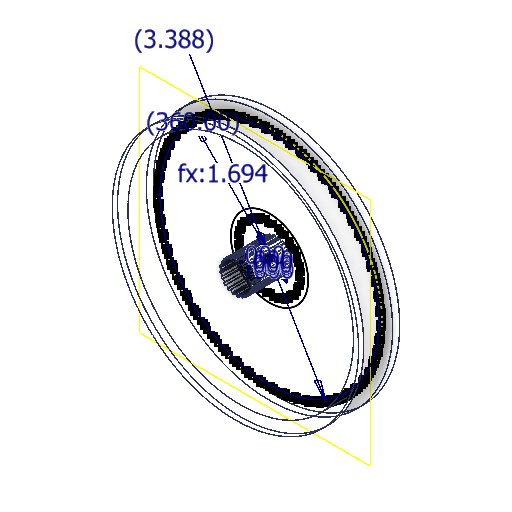
# Autodesk Inventor part: Diff Large Pulley
Saved by Autodesk Inventor 2025.2 (Build 292293000, 293)
## iProperties
Created: 2025-02-20
Part Number: Diff Large Pulley
Material: Generic
Document SubType Name: Modeling
Designer: Jakeg
Density: 1 g/cm^3
Appearance: PTFE
Author: Jakeg
Autodesk Inventor part; units mm, degrees
(part 1 of 2)
ref_plane "YZ Plane" through (0, 0, 0) normal (1, 0, 0) x (0, 1, 0)
ref_plane "XZ Plane" through (0, 0, 0) normal (0, 1, 0) x (-1, 0, 0)
ref_plane "XY Plane" through (0, 0, 0) normal (0, 0, 1) x (1, 0, 0)
sketch "Sketch1" plane through (0, 0, 0) normal (0, 0, 1) x (1, 0, 0)
  circle A0 centre (0, 0) radius 46.99
  dimension "d0" = 93.98
  constraints: 1 centre point, 1 coincident
  measures "d0" diameter of A0
extrude "Extrusion1" add sketch "Sketch1" along normal blind 15.7
ref_plane "Work Plane1" through (0, 0, 8.2) normal (0, 0, 1) x (1, 0, 0)
sketch "Sketch2" plane through (0, 0, 8.2) normal (0, 0, 1) x (1, 0, 0)
  circle A0 centre (0, 0) radius 43.0276
  circle A1 centre (0, 0) radius 46.99
  dimension "d4" = 86.0552
  dimension "d39" = 93.98
  constraints: 2 centre point, 2 coincident
  measures "d4" diameter of A0
  measures "d39" diameter of A1
extrude "Extrusion2" cut sketch "Sketch2" along normal mid plane 11
sketch "Sketch3" plane through (0, 0, 15.7) normal (0, 0, 1) x (1, 0, 0)
  circle A0 centre (0, 0) radius 6
  circle A1 centre (0, 20.32) radius 3.175
  circle A2 centre (0, -20.32) radius 3.175
  dimension "d7" = 12
  dimension "d13" = 6.35
  dimension "d14" = 20.32
  dimension "d15" = 6.35
  dimension "d16" = 20.32
  constraints: 3 centre point, 1 coincident
  measures "d7" diameter of A0
  measures "d13" diameter of A1
  measures "d14" distance of point (0, 0) A1.centre
  measures "d15" diameter of A2
  measures "d16" distance of point (0, 0) A2.centre
extrude "Extrusion3" cut sketch "Sketch3" against normal through all contours A0
sketch "Sketch5" plane through (0, 0, 15.7) normal (0, 0, 1) x (1, 0, 0)
  circle A0 centre (0, 0) radius 6 projected
  arc A1 (-1.2778, -5.5469) -> (-2.2267, -5.2386) centre (-1.8274, -5.6241) ccw
  arc A2 (-1.2783, -5.8289) -> (-1.2778, -5.5469) centre (-2.2681, -5.6859) ccw
  arc A3 (-1.2783, -5.8289) -> (-1.1583, -5.9977) centre (-1.1299, -5.8504) ccw
  arc A4 (-1.1583, -5.9977) -> (-0.7518, -6.0621) centre (0, 0) ccw
  arc A5 (-0.7518, -6.0621) -> (-0.5855, -5.9387) centre (-0.7333, -5.9132) ccw
  arc A6 (-0.4989, -5.6703) -> (-0.5855, -5.9387) centre (0.4, -6.1085) ccw
  arc A7 (0.4989, -5.6703) -> (-0.4989, -5.6703) centre (0, -5.9135) ccw
  arc A8 (0.5855, -5.9387) -> (0.4989, -5.6703) centre (-0.4, -6.1085) ccw
  arc A9 (0.5855, -5.9387) -> (0.7518, -6.0621) centre (0.7333, -5.9132) ccw
  arc A10 (0.7518, -6.0621) -> (1.1583, -5.9977) centre (0, 0) ccw
  arc A11 (1.1583, -5.9977) -> (1.2783, -5.8289) centre (1.1299, -5.8504) ccw
  arc A12 (1.2778, -5.5469) -> (1.2783, -5.8289) centre (2.2681, -5.6859) ccw
  arc A13 (2.2267, -5.2386) -> (1.2778, -5.5469) centre (1.8274, -5.6241) ccw
  arc A14 (2.392, -5.4671) -> (2.2267, -5.2386) centre (1.5072, -5.9331) ccw
  arc A15 (2.392, -5.4671) -> (2.5882, -5.5331) centre (2.5247, -5.3972) ccw
  arc A16 (2.5882, -5.5331) -> (2.955, -5.3462) centre (0, 0) ccw
  arc A17 (2.955, -5.3462) -> (3.017, -5.1486) centre (2.8824, -5.2149) ccw
  arc A18 (2.9293, -4.8806) -> (3.017, -5.1486) centre (3.9141, -4.7068) ccw
  arc A19 (3.7365, -4.2941) -> (2.9293, -4.8806) centre (3.4759, -4.7841) ccw
  arc A20 (3.9643, -4.4604) -> (3.7365, -4.2941) centre (3.2669, -5.177) ccw
  arc A21 (3.9643, -4.4604) -> (4.1714, -4.4624) centre (4.0689, -4.3529) ccw
  arc A22 (4.1714, -4.4624) -> (4.4624, -4.1714) centre (0, 0) ccw
  arc A23 (4.4624, -4.1714) -> (4.4604, -3.9643) centre (4.3529, -4.0689) ccw
  arc A24 (4.2941, -3.7365) -> (4.4604, -3.9643) centre (5.177, -3.2669) ccw
  arc A25 (4.8806, -2.9293) -> (4.2941, -3.7365) centre (4.7841, -3.4759) ccw
  arc A26 (5.1486, -3.017) -> (4.8806, -2.9293) centre (4.7068, -3.9141) ccw
  arc A27 (5.1486, -3.017) -> (5.3462, -2.955) centre (5.2149, -2.8824) ccw
  arc A28 (5.3462, -2.955) -> (5.5331, -2.5882) centre (0, 0) ccw
  arc A29 (5.5331, -2.5882) -> (5.4671, -2.392) centre (5.3972, -2.5247) ccw
  arc A30 (5.2386, -2.2267) -> (5.4671, -2.392) centre (5.9331, -1.5072) ccw
  arc A31 (5.5469, -1.2778) -> (5.2386, -2.2267) centre (5.6241, -1.8274) ccw
  arc A32 (5.8289, -1.2783) -> (5.5469, -1.2778) centre (5.6859, -2.2681) ccw
  arc A33 (5.8289, -1.2783) -> (5.9977, -1.1583) centre (5.8504, -1.1299) ccw
  arc A34 (5.9977, -1.1583) -> (6.0621, -0.7518) centre (0, 0) ccw
  arc A35 (6.0621, -0.7518) -> (5.9387, -0.5855) centre (5.9132, -0.7333) ccw
  arc A36 (5.6703, -0.4989) -> (5.9387, -0.5855) centre (6.1085, 0.4) ccw
  arc A37 (5.6703, 0.4989) -> (5.6703, -0.4989) centre (5.9135, 0) ccw
  arc A38 (5.9387, 0.5855) -> (5.6703, 0.4989) centre (6.1085, -0.4) ccw
  arc A39 (5.9387, 0.5855) -> (6.0621, 0.7518) centre (5.9132, 0.7333) ccw
  arc A40 (6.0621, 0.7518) -> (5.9977, 1.1583) centre (0, 0) ccw
  arc A41 (5.9977, 1.1583) -> (5.8289, 1.2783) centre (5.8504, 1.1299) ccw
  arc A42 (5.5469, 1.2778) -> (5.8289, 1.2783) centre (5.6859, 2.2681) ccw
  arc A43 (5.2386, 2.2267) -> (5.5469, 1.2778) centre (5.6241, 1.8274) ccw
  arc A44 (5.4671, 2.392) -> (5.2386, 2.2267) centre (5.9331, 1.5072) ccw
  arc A45 (5.4671, 2.392) -> (5.5331, 2.5882) centre (5.3972, 2.5247) ccw
  arc A46 (5.5331, 2.5882) -> (5.3462, 2.955) centre (0, 0) ccw
  arc A47 (5.3462, 2.955) -> (5.1486, 3.017) centre (5.2149, 2.8824) ccw
  arc A48 (4.8806, 2.9293) -> (5.1486, 3.017) centre (4.7068, 3.9141) ccw
  arc A49 (4.2941, 3.7365) -> (4.8806, 2.9293) centre (4.7841, 3.4759) ccw
  arc A50 (4.4604, 3.9643) -> (4.2941, 3.7365) centre (5.177, 3.2669) ccw
  arc A51 (4.4604, 3.9643) -> (4.4624, 4.1714) centre (4.3529, 4.0689) ccw
  arc A52 (4.4624, 4.1714) -> (4.1714, 4.4624) centre (0, 0) ccw
  arc A53 (4.1714, 4.4624) -> (3.9643, 4.4604) centre (4.0689, 4.3529) ccw
  arc A54 (3.7365, 4.2941) -> (3.9643, 4.4604) centre (3.2669, 5.177) ccw
  arc A55 (2.9293, 4.8806) -> (3.7365, 4.2941) centre (3.4759, 4.7841) ccw
  arc A56 (3.017, 5.1486) -> (2.9293, 4.8806) centre (3.9141, 4.7068) ccw
  arc A57 (3.017, 5.1486) -> (2.955, 5.3462) centre (2.8824, 5.2149) ccw
  arc A58 (2.955, 5.3462) -> (2.5882, 5.5331) centre (0, 0) ccw
  arc A59 (2.5882, 5.5331) -> (2.392, 5.4671) centre (2.5247, 5.3972) ccw
  arc A60 (2.2267, 5.2386) -> (2.392, 5.4671) centre (1.5072, 5.9331) ccw
  arc A61 (1.2778, 5.5469) -> (2.2267, 5.2386) centre (1.8274, 5.6241) ccw
  arc A62 (1.2783, 5.8289) -> (1.2778, 5.5469) centre (2.2681, 5.6859) ccw
  arc A63 (1.2783, 5.8289) -> (1.1583, 5.9977) centre (1.1299, 5.8504) ccw
  arc A64 (1.1583, 5.9977) -> (0.7518, 6.0621) centre (0, 0) ccw
  arc A65 (0.7518, 6.0621) -> (0.5855, 5.9387) centre (0.7333, 5.9132) ccw
  arc A66 (0.4989, 5.6703) -> (0.5855, 5.9387) centre (-0.4, 6.1085) ccw
  arc A67 (-0.4989, 5.6703) -> (0.4989, 5.6703) centre (0, 5.9135) ccw
  arc A68 (-0.5855, 5.9387) -> (-0.4989, 5.6703) centre (0.4, 6.1085) ccw
  arc A69 (-0.5855, 5.9387) -> (-0.7518, 6.0621) centre (-0.7333, 5.9132) ccw
  arc A70 (-0.7518, 6.0621) -> (-1.1583, 5.9977) centre (0, 0) ccw
  arc A71 (-1.1583, 5.9977) -> (-1.2783, 5.8289) centre (-1.1299, 5.8504) ccw
  arc A72 (-1.2778, 5.5469) -> (-1.2783, 5.8289) centre (-2.2681, 5.6859) ccw
  arc A73 (-2.2267, 5.2386) -> (-1.2778, 5.5469) centre (-1.8274, 5.6241) ccw
  arc A74 (-2.392, 5.4671) -> (-2.2267, 5.2386) centre (-1.5072, 5.9331) ccw
  arc A75 (-2.392, 5.4671) -> (-2.5882, 5.5331) centre (-2.5247, 5.3972) ccw
  arc A76 (-2.5882, 5.5331) -> (-2.955, 5.3462) centre (0, 0) ccw
  arc A77 (-2.955, 5.3462) -> (-3.017, 5.1486) centre (-2.8824, 5.2149) ccw
  arc A78 (-2.9293, 4.8806) -> (-3.017, 5.1486) centre (-3.9141, 4.7068) ccw
  arc A79 (-3.7365, 4.2941) -> (-2.9293, 4.8806) centre (-3.4759, 4.7841) ccw
  arc A80 (-3.9643, 4.4604) -> (-3.7365, 4.2941) centre (-3.2669, 5.177) ccw
  arc A81 (-3.9643, 4.4604) -> (-4.1714, 4.4624) centre (-4.0689, 4.3529) ccw
  arc A82 (-4.1714, 4.4624) -> (-4.4624, 4.1714) centre (0, 0) ccw
  arc A83 (-4.4624, 4.1714) -> (-4.4604, 3.9643) centre (-4.3529, 4.0689) ccw
  arc A84 (-4.2941, 3.7365) -> (-4.4604, 3.9643) centre (-5.177, 3.2669) ccw
  arc A85 (-4.8806, 2.9293) -> (-4.2941, 3.7365) centre (-4.7841, 3.4759) ccw
  arc A86 (-5.1486, 3.017) -> (-4.8806, 2.9293) centre (-4.7068, 3.9141) ccw
  arc A87 (-5.1486, 3.017) -> (-5.3462, 2.955) centre (-5.2149, 2.8824) ccw
  arc A88 (-5.3462, 2.955) -> (-5.5331, 2.5882) centre (0, 0) ccw
  arc A89 (-5.5331, 2.5882) -> (-5.4671, 2.392) centre (-5.3972, 2.5247) ccw
  arc A90 (-5.2386, 2.2267) -> (-5.4671, 2.392) centre (-5.9331, 1.5072) ccw
  arc A91 (-5.5469, 1.2778) -> (-5.2386, 2.2267) centre (-5.6241, 1.8274) ccw
  arc A92 (-5.8289, 1.2783) -> (-5.5469, 1.2778) centre (-5.6859, 2.2681) ccw
  arc A93 (-5.8289, 1.2783) -> (-5.9977, 1.1583) centre (-5.8504, 1.1299) ccw
  arc A94 (-5.9977, 1.1583) -> (-6.0621, 0.7518) centre (0, 0) ccw
  arc A95 (-6.0621, 0.7518) -> (-5.9387, 0.5855) centre (-5.9132, 0.7333) ccw
  arc A96 (-5.6703, 0.4989) -> (-5.9387, 0.5855) centre (-6.1085, -0.4) ccw
  arc A97 (-5.6703, -0.4989) -> (-5.6703, 0.4989) centre (-5.9135, 0) ccw
  arc A98 (-5.9387, -0.5855) -> (-5.6703, -0.4989) centre (-6.1085, 0.4) ccw
  arc A99 (-5.9387, -0.5855) -> (-6.0621, -0.7518) centre (-5.9132, -0.7333) ccw
  arc A100 (-6.0621, -0.7518) -> (-5.9977, -1.1583) centre (0, 0) ccw
  arc A101 (-5.9977, -1.1583) -> (-5.8289, -1.2783) centre (-5.8504, -1.1299) ccw
  arc A102 (-5.5469, -1.2778) -> (-5.8289, -1.2783) centre (-5.6859, -2.2681) ccw
  arc A103 (-5.2386, -2.2267) -> (-5.5469, -1.2778) centre (-5.6241, -1.8274) ccw
  arc A104 (-5.4671, -2.392) -> (-5.2386, -2.2267) centre (-5.9331, -1.5072) ccw
  arc A105 (-5.4671, -2.392) -> (-5.5331, -2.5882) centre (-5.3972, -2.5247) ccw
  arc A106 (-5.5331, -2.5882) -> (-5.3462, -2.955) centre (0, 0) ccw
  arc A107 (-5.3462, -2.955) -> (-5.1486, -3.017) centre (-5.2149, -2.8824) ccw
  arc A108 (-4.8806, -2.9293) -> (-5.1486, -3.017) centre (-4.7068, -3.9141) ccw
  arc A109 (-4.2941, -3.7365) -> (-4.8806, -2.9293) centre (-4.7841, -3.4759) ccw
  arc A110 (-4.4604, -3.9643) -> (-4.2941, -3.7365) centre (-5.177, -3.2669) ccw
  arc A111 (-4.4604, -3.9643) -> (-4.4624, -4.1714) centre (-4.3529, -4.0689) ccw
  arc A112 (-4.4624, -4.1714) -> (-4.1714, -4.4624) centre (0, 0) ccw
  arc A113 (-4.1714, -4.4624) -> (-3.9643, -4.4604) centre (-4.0689, -4.3529) ccw
  arc A114 (-3.7365, -4.2941) -> (-3.9643, -4.4604) centre (-3.2669, -5.177) ccw
  arc A115 (-2.9293, -4.8806) -> (-3.7365, -4.2941) centre (-3.4759, -4.7841) ccw
  arc A116 (-3.017, -5.1486) -> (-2.9293, -4.8806) centre (-3.9141, -4.7068) ccw
  arc A117 (-3.017, -5.1486) -> (-2.955, -5.3462) centre (-2.8824, -5.2149) ccw
  arc A118 (-2.955, -5.3462) -> (-2.5882, -5.5331) centre (0, 0) ccw
  arc A119 (-2.5882, -5.5331) -> (-2.392, -5.4671) centre (-2.5247, -5.3972) ccw
  arc A120 (-2.2267, -5.2386) -> (-2.392, -5.4671) centre (-1.5072, -5.9331) ccw
  point P0 (-3.9904, -4.4807)
  point P1 (-3.0283, -5.1797)
  point P2 (-5.1797, -3.0283)
  point P3 (-4.4807, -3.9904)
  point P4 (-5.862, -1.2794)
  point P5 (-5.4945, -2.4105)
  point P6 (-5.9705, 0.5947)
  point P7 (-5.9705, -0.5947)
  point P8 (-5.4945, 2.4105)
  point P9 (-5.862, 1.2794)
  point P10 (-4.4807, 3.9904)
  point P11 (-5.1797, 3.0283)
  point P12 (-3.0283, 5.1797)
  point P13 (-3.9904, 4.4807)
  point P14 (-1.2794, 5.862)
  point P15 (-2.4105, 5.4945)
  point P16 (0.5947, 5.9705)
  point P17 (-0.5947, 5.9705)
  point P18 (2.4105, 5.4945)
  point P19 (1.2794, 5.862)
  point P20 (3.9904, 4.4807)
  point P21 (3.0283, 5.1797)
  point P22 (5.1797, 3.0283)
  point P23 (4.4807, 3.9904)
  point P24 (5.862, 1.2794)
  point P25 (5.4945, 2.4105)
  point P26 (5.9705, -0.5947)
  point P27 (5.9705, 0.5947)
  point P28 (5.4945, -2.4105)
  point P29 (5.862, -1.2794)
  point P30 (4.4807, -3.9904)
  point P31 (5.1797, -3.0283)
  point P32 (3.0283, -5.1797)
  point P33 (3.9904, -4.4807)
  point P34 (1.2794, -5.862)
  point P35 (2.4105, -5.4945)
  point P36 (-0.5947, -5.9705)
  point P37 (0.5947, -5.9705)
  point P38 (-2.4105, -5.4945)
  point P39 (-1.2794, -5.862)
  dimension "d21" = 0
  dimension "d22" = 0
  constraints: 240 point on circle, 120 centre point, 1 coincident, 1 other
  measures "d21" distance of point (0, 0) A4.centre
  measures "d22" distance of A4.centre point (0, 0)
extrude "Extrusion5" add sketch "Sketch5" against normal blind 15.7 contours A0 A35 A36 A37 A38 A39 | A0 A41 A40 A39 | A35 A34 A33 A0 | A41 A42 A43 A44 A45 A0 | A0 A29 A30 A31 A32 A33 | A0 A47 A46 A45 | A29 A28 A27 A0 | A47 A48 A49 A50 A51 A0 | A0 A23 A24 A25 A26 A27 | A0 A53 A52 A51 | A23 A22 A21 A0 | A53 A54 A55 A56 A57 A0 | A0 A17 A18 A19 A20 A21 | A0 A59 A58 A57 | A17 A16 A15 A0 | A59 A60 A61 A62 A63 A0 | A0 A11 A12 A13 A14 A15 | A0 A65 A64 A63 | A11 A10 A9 A0 | A65 A66 A67 A68 A69 A0 | A0 A5 A6 A7 A8 A9 | A0 A71 A70 A69 | A5 A4 A3 A0 | A71 A72 A73 A74 A75 A0 | A0 A119 A120 A1 A2 A3 | A0 A77 A76 A75 | A119 A118 A117 A0 | A77 A78 A79 A80 A81 A0 | A0 A113 A114 A115 A116 A117 | A0 A83 A82 A81 | A113 A112 A111 A0 | A83 A84 A85 A86 A87 A0 | A0 A107 A108 A109 A110 A111 | A0 A89 A88 A87 | A107 A106 A105 A0 | A89 A90 A91 A92 A93 A0 | A0 A101 A102 A103 A104 A105 | A0 A95 A94 A93 | A101 A100 A99 A0 | A95 A96 A97 A98 A99 A0
sketch "Sketch8" plane through (0, 0, 2.7) normal (0, 0, 1) x (1, 0, 0)
  circle A0 centre (0, 0) radius 14.7498
  line L0 (3.5809, 11.7957) -> (3.627, 10.7394)
  arc A1 (3.627, 10.7394) -> (3.7836, 10.5159) centre (3.8808, 10.7505) ccw
  line L1 (3.7836, 10.5159) -> (4.7604, 10.1112)
  arc A2 (4.7604, 10.1112) -> (5.0292, 10.1586) centre (4.8576, 10.3459) ccw
  line L2 (5.0292, 10.1586) -> (5.8087, 10.8729)
  arc A3 (6.1044, 10.9073) -> (5.8087, 10.8729) centre (5.9803, 10.6856) ccw
  arc A4 (7.741, 9.8138) -> (6.1044, 10.9073) centre (0, 0) ccw
  arc A5 (7.8223, 9.5275) -> (7.741, 9.8138) centre (7.5837, 9.6143) ccw
  line L3 (7.8223, 9.5275) -> (7.4607, 8.534)
  arc A6 (7.4607, 8.534) -> (7.5198, 8.2675) centre (7.6994, 8.4471) ccw
  line L4 (7.5198, 8.2675) -> (8.2675, 7.5198)
  arc A7 (8.2675, 7.5198) -> (8.534, 7.4607) centre (8.4471, 7.6994) ccw
  line L5 (8.534, 7.4607) -> (9.5275, 7.8223)
  arc A8 (9.8138, 7.741) -> (9.5275, 7.8223) centre (9.6143, 7.5837) ccw
  arc A9 (10.9073, 6.1044) -> (9.8138, 7.741) centre (0, 0) ccw
  arc A10 (10.8729, 5.8087) -> (10.9073, 6.1044) centre (10.6856, 5.9803) ccw
  line L6 (10.8729, 5.8087) -> (10.1586, 5.0292)
  arc A11 (10.1586, 5.0292) -> (10.1112, 4.7604) centre (10.3459, 4.8576) ccw
  line L7 (10.1112, 4.7604) -> (10.5159, 3.7836)
  arc A12 (10.5159, 3.7836) -> (10.7394, 3.627) centre (10.7505, 3.8808) ccw
  line L8 (10.7394, 3.627) -> (11.7957, 3.5809)
  arc A13 (12.0291, 3.3962) -> (11.7957, 3.5809) centre (11.7846, 3.3271) ccw
  arc A14 (12.4131, 1.4657) -> (12.0291, 3.3962) centre (0, 0) ccw
  arc A15 (12.2682, 1.2057) -> (12.4131, 1.4657) centre (12.1608, 1.4359) ccw
  line L9 (12.2682, 1.2057) -> (11.31, 0.7589)
  arc A16 (11.31, 0.7589) -> (11.1633, 0.5287) centre (11.4173, 0.5287) ccw
  line L10 (11.1633, 0.5287) -> (11.1633, -0.5287)
  arc A17 (11.1633, -0.5287) -> (11.31, -0.7589) centre (11.4173, -0.5287) ccw
  line L11 (11.31, -0.7589) -> (12.2682, -1.2057)
  arc A18 (12.4131, -1.4657) -> (12.2682, -1.2057) centre (12.1608, -1.4359) ccw
  arc A19 (12.0291, -3.3962) -> (12.4131, -1.4657) centre (0, 0) ccw
  arc A20 (11.7957, -3.5809) -> (12.0291, -3.3962) centre (11.7846, -3.3271) ccw
  line L12 (11.7957, -3.5809) -> (10.7394, -3.627)
  arc A21 (10.7394, -3.627) -> (10.5159, -3.7836) centre (10.7505, -3.8808) ccw
  line L13 (10.5159, -3.7836) -> (10.1112, -4.7604)
  arc A22 (10.1112, -4.7604) -> (10.1586, -5.0292) centre (10.3459, -4.8576) ccw
  line L14 (10.1586, -5.0292) -> (10.8729, -5.8087)
  arc A23 (10.9073, -6.1044) -> (10.8729, -5.8087) centre (10.6856, -5.9803) ccw
  arc A24 (9.8138, -7.741) -> (10.9073, -6.1044) centre (0, 0) ccw
  arc A25 (9.5275, -7.8223) -> (9.8138, -7.741) centre (9.6143, -7.5837) ccw
  line L15 (9.5275, -7.8223) -> (8.534, -7.4607)
  arc A26 (8.534, -7.4607) -> (8.2675, -7.5198) centre (8.4471, -7.6994) ccw
  line L16 (8.2675, -7.5198) -> (7.5198, -8.2675)
  arc A27 (7.5198, -8.2675) -> (7.4607, -8.534) centre (7.6994, -8.4471) ccw
  line L17 (7.4607, -8.534) -> (7.8223, -9.5275)
  arc A28 (7.741, -9.8138) -> (7.8223, -9.5275) centre (7.5837, -9.6143) ccw
  arc A29 (6.1044, -10.9073) -> (7.741, -9.8138) centre (0, 0) ccw
  arc A30 (5.8087, -10.8729) -> (6.1044, -10.9073) centre (5.9803, -10.6856) ccw
  line L18 (5.8087, -10.8729) -> (5.0292, -10.1586)
  arc A31 (5.0292, -10.1586) -> (4.7604, -10.1112) centre (4.8576, -10.3459) ccw
  line L19 (4.7604, -10.1112) -> (3.7836, -10.5159)
  arc A32 (3.7836, -10.5159) -> (3.627, -10.7394) centre (3.8808, -10.7505) ccw
  line L20 (3.627, -10.7394) -> (3.5809, -11.7957)
  arc A33 (3.3962, -12.0291) -> (3.5809, -11.7957) centre (3.3271, -11.7846) ccw
  arc A34 (1.4657, -12.4131) -> (3.3962, -12.0291) centre (0, 0) ccw
  arc A35 (1.2057, -12.2682) -> (1.4657, -12.4131) centre (1.4359, -12.1608) ccw
  line L21 (1.2057, -12.2682) -> (0.7589, -11.31)
  arc A36 (0.7589, -11.31) -> (0.5287, -11.1633) centre (0.5287, -11.4173) ccw
  line L22 (0.5287, -11.1633) -> (-0.5287, -11.1633)
  arc A37 (-0.5287, -11.1633) -> (-0.7589, -11.31) centre (-0.5287, -11.4173) ccw
  line L23 (-0.7589, -11.31) -> (-1.2057, -12.2682)
  arc A38 (-1.4657, -12.4131) -> (-1.2057, -12.2682) centre (-1.4359, -12.1608) ccw
  arc A39 (-3.3962, -12.0291) -> (-1.4657, -12.4131) centre (0, 0) ccw
  arc A40 (-3.5809, -11.7957) -> (-3.3962, -12.0291) centre (-3.3271, -11.7846) ccw
  line L24 (-3.5809, -11.7957) -> (-3.627, -10.7394)
  arc A41 (-3.627, -10.7394) -> (-3.7836, -10.5159) centre (-3.8808, -10.7505) ccw
  line L25 (-3.7836, -10.5159) -> (-4.7604, -10.1112)
  arc A42 (-4.7604, -10.1112) -> (-5.0292, -10.1586) centre (-4.8576, -10.3459) ccw
  line L26 (-5.0292, -10.1586) -> (-5.8087, -10.8729)
  arc A43 (-6.1044, -10.9073) -> (-5.8087, -10.8729) centre (-5.9803, -10.6856) ccw
  arc A44 (-7.741, -9.8138) -> (-6.1044, -10.9073) centre (0, 0) ccw
  arc A45 (-7.8223, -9.5275) -> (-7.741, -9.8138) centre (-7.5837, -9.6143) ccw
  line L27 (-7.8223, -9.5275) -> (-7.4607, -8.534)
  arc A46 (-7.4607, -8.534) -> (-7.5198, -8.2675) centre (-7.6994, -8.4471) ccw
  line L28 (-7.5198, -8.2675) -> (-8.2675, -7.5198)
  arc A47 (-8.2675, -7.5198) -> (-8.534, -7.4607) centre (-8.4471, -7.6994) ccw
  line L29 (-8.534, -7.4607) -> (-9.5275, -7.8223)
  arc A48 (-9.8138, -7.741) -> (-9.5275, -7.8223) centre (-9.6143, -7.5837) ccw
  arc A49 (-10.9073, -6.1044) -> (-9.8138, -7.741) centre (0, 0) ccw
  arc A50 (-10.8729, -5.8087) -> (-10.9073, -6.1044) centre (-10.6856, -5.9803) ccw
  line L30 (-10.8729, -5.8087) -> (-10.1586, -5.0292)
  arc A51 (-10.1586, -5.0292) -> (-10.1112, -4.7604) centre (-10.3459, -4.8576) ccw
  line L31 (-10.1112, -4.7604) -> (-10.5159, -3.7836)
  arc A52 (-10.5159, -3.7836) -> (-10.7394, -3.627) centre (-10.7505, -3.8808) ccw
  line L32 (-10.7394, -3.627) -> (-11.7957, -3.5809)
  arc A53 (-12.0291, -3.3962) -> (-11.7957, -3.5809) centre (-11.7846, -3.3271) ccw
  arc A54 (-12.4131, -1.4657) -> (-12.0291, -3.3962) centre (0, 0) ccw
  arc A55 (-12.2682, -1.2057) -> (-12.4131, -1.4657) centre (-12.1608, -1.4359) ccw
  line L33 (-12.2682, -1.2057) -> (-11.31, -0.7589)
  arc A56 (-11.31, -0.7589) -> (-11.1633, -0.5287) centre (-11.4173, -0.5287) ccw
  line L34 (-11.1633, -0.5287) -> (-11.1633, 0.5287)
  arc A57 (-11.1633, 0.5287) -> (-11.31, 0.7589) centre (-11.4173, 0.5287) ccw
  line L35 (-11.31, 0.7589) -> (-12.2682, 1.2057)
  arc A58 (-12.4131, 1.4657) -> (-12.2682, 1.2057) centre (-12.1608, 1.4359) ccw
  arc A59 (-12.0291, 3.3962) -> (-12.4131, 1.4657) centre (0, 0) ccw
  arc A60 (-11.7957, 3.5809) -> (-12.0291, 3.3962) centre (-11.7846, 3.3271) ccw
  line L36 (-11.7957, 3.5809) -> (-10.7394, 3.627)
  arc A61 (-10.7394, 3.627) -> (-10.5159, 3.7836) centre (-10.7505, 3.8808) ccw
  line L37 (-10.5159, 3.7836) -> (-10.1112, 4.7604)
  arc A62 (-10.1112, 4.7604) -> (-10.1586, 5.0292) centre (-10.3459, 4.8576) ccw
  line L38 (-10.1586, 5.0292) -> (-10.8729, 5.8087)
  arc A63 (-10.9073, 6.1044) -> (-10.8729, 5.8087) centre (-10.6856, 5.9803) ccw
  arc A64 (-9.8138, 7.741) -> (-10.9073, 6.1044) centre (0, 0) ccw
  arc A65 (-9.5275, 7.8223) -> (-9.8138, 7.741) centre (-9.6143, 7.5837) ccw
  line L39 (-9.5275, 7.8223) -> (-8.534, 7.4607)
  arc A66 (-8.534, 7.4607) -> (-8.2675, 7.5198) centre (-8.4471, 7.6994) ccw
  line L40 (-8.2675, 7.5198) -> (-7.5198, 8.2675)
  arc A67 (-7.5198, 8.2675) -> (-7.4607, 8.534) centre (-7.6994, 8.4471) ccw
  line L41 (-7.4607, 8.534) -> (-7.8223, 9.5275)
  arc A68 (-7.741, 9.8138) -> (-7.8223, 9.5275) centre (-7.5837, 9.6143) ccw
  arc A69 (-6.1044, 10.9073) -> (-7.741, 9.8138) centre (0, 0) ccw
  arc A70 (-5.8087, 10.8729) -> (-6.1044, 10.9073) centre (-5.9803, 10.6856) ccw
  line L42 (-5.8087, 10.8729) -> (-5.0292, 10.1586)
  arc A71 (-5.0292, 10.1586) -> (-4.7604, 10.1112) centre (-4.8576, 10.3459) ccw
  line L43 (-4.7604, 10.1112) -> (-3.7836, 10.5159)
  arc A72 (-3.7836, 10.5159) -> (-3.627, 10.7394) centre (-3.8808, 10.7505) ccw
  line L44 (-3.627, 10.7394) -> (-3.5809, 11.7957)
  arc A73 (-3.3962, 12.0291) -> (-3.5809, 11.7957) centre (-3.3271, 11.7846) ccw
  arc A74 (-1.4657, 12.4131) -> (-3.3962, 12.0291) centre (0, 0) ccw
  arc A75 (-1.2057, 12.2682) -> (-1.4657, 12.4131) centre (-1.4359, 12.1608) ccw
  line L45 (-1.2057, 12.2682) -> (-0.7589, 11.31)
  arc A76 (-0.7589, 11.31) -> (-0.5287, 11.1633) centre (-0.5287, 11.4173) ccw
  line L46 (-0.5287, 11.1633) -> (0.5287, 11.1633)
  arc A77 (0.5287, 11.1633) -> (0.7589, 11.31) centre (0.5287, 11.4173) ccw
  line L47 (0.7589, 11.31) -> (1.2057, 12.2682)
  arc A78 (1.4657, 12.4131) -> (1.2057, 12.2682) centre (1.4359, 12.1608) ccw
  arc A79 (3.3962, 12.0291) -> (1.4657, 12.4131) centre (0, 0) ccw
  arc A80 (3.5809, 11.7957) -> (3.3962, 12.0291) centre (3.3271, 11.7846) ccw
  circle A81 centre (0, 0) radius 43.0276 projected
  arc A82 (-31.1752, 29.4701) -> (-31.4615, 29.3887) centre (-31.2621, 29.2314) ccw
  line L48 (-31.1752, 29.4701) -> (-30.1817, 29.1085)
  arc A83 (-30.1817, 29.1085) -> (-29.9152, 29.1676) centre (-30.0948, 29.3472) ccw
  line L49 (-29.9152, 29.1676) -> (-29.1676, 29.9152)
  arc A84 (-29.1676, 29.9152) -> (-29.1085, 30.1817) centre (-29.3472, 30.0948) ccw
  line L50 (-29.1085, 30.1817) -> (-29.4701, 31.1752)
  arc A85 (-29.3887, 31.4615) -> (-29.4701, 31.1752) centre (-29.2314, 31.2621) ccw
  circle A86 centre (0, 0) radius 43.0276
  line L51 (-31.4615, 29.3887) -> (-29.3887, 31.4615)
  arc A87 (-32.231, 26.5863) -> (-32.2011, 26.8576) centre (-32.429, 26.7454) ccw
  arc A88 (-33.152, 25.6746) -> (-32.8934, 25.7622) centre (-33.0914, 25.9213) ccw
  line L52 (-32.2011, 26.8576) -> (-32.668, 27.8062)
  line L53 (-34.1787, 25.9267) -> (-33.152, 25.6746)
  line L54 (-32.8934, 25.7622) -> (-32.231, 26.5863)
  arc A89 (-34.1787, 25.9267) -> (-34.4545, 25.8149) centre (-34.2393, 25.68) ccw
  line L55 (-34.4545, 25.8149) -> (-32.618, 28.0996)
  arc A90 (-32.618, 28.0996) -> (-32.668, 27.8062) centre (-32.4401, 27.9183) ccw
  arc A91 (-34.9165, 22.9457) -> (-34.9161, 23.2186) centre (-35.1305, 23.0825) ccw
  arc A92 (-35.7335, 21.9398) -> (-35.486, 22.0548) centre (-35.7, 22.1916) ccw
  line L56 (-34.9161, 23.2186) -> (-35.4828, 24.1111)
  line L57 (-36.7815, 22.0794) -> (-35.7335, 21.9398)
  line L58 (-35.486, 22.0548) -> (-34.9165, 22.9457)
  arc A93 (-36.7815, 22.0794) -> (-37.0437, 21.9383) centre (-36.8151, 21.8276) ccw
  line L59 (-37.0437, 21.9383) -> (-35.4649, 24.4082)
  arc A94 (-35.4649, 24.4082) -> (-35.4828, 24.1111) centre (-35.2684, 24.2473) ccw
  arc A95 (-37.1927, 19.036) -> (-37.2218, 19.3074) centre (-37.4203, 19.1489) ccw
  arc A96 (-37.8962, 17.9477) -> (-37.6625, 18.0888) centre (-37.8901, 18.2016) ccw
  line L60 (-37.2218, 19.3074) -> (-37.8817, 20.1334)
  line L61 (-38.9531, 17.9731) -> (-37.8962, 17.9477)
  line L62 (-37.6625, 18.0888) -> (-37.1927, 19.036)
  arc A97 (-38.9531, 17.9731) -> (-39.1985, 17.8046) centre (-38.9592, 17.7192) ccw
  line L63 (-39.1985, 17.8046) -> (-37.896, 20.4307)
  arc A98 (-37.896, 20.4307) -> (-37.8817, 20.1334) centre (-37.6833, 20.292) ccw
  arc A99 (-39.0328, 14.9032) -> (-39.0911, 15.1698) centre (-39.2713, 14.9908) ccw
  arc A100 (-39.6145, 13.7452) -> (-39.3975, 13.9107) centre (-39.6359, 13.9983) ccw
  line L64 (-39.0911, 15.1698) -> (-39.8365, 15.9197)
  line L65 (-40.668, 13.6562) -> (-39.6145, 13.7452)
  line L66 (-39.3975, 13.9107) -> (-39.0328, 14.9032)
  arc A101 (-40.668, 13.6562) -> (-40.8937, 13.4621) centre (-40.6466, 13.4031) ccw
  line L67 (-40.8937, 13.4621) -> (-39.8828, 16.2137)
  arc A102 (-39.8828, 16.2137) -> (-39.8365, 15.9197) centre (-39.6563, 16.0987) ccw
  arc A103 (-40.4153, 10.5956) -> (-40.5021, 10.8544) centre (-40.6618, 10.6569) ccw
  arc A104 (-40.8684, 9.3815) -> (-40.6705, 9.5695) centre (-40.917, 9.6308) ccw
  line L68 (-40.5021, 10.8544) -> (-41.3242, 11.5193)
  line L69 (-41.9061, 9.1792) -> (-40.8684, 9.3815)
  line L70 (-40.6705, 9.5695) -> (-40.4153, 10.5956)
  arc A105 (-41.9061, 9.1792) -> (-42.1095, 8.9618) centre (-41.8575, 8.9299) ccw
  line L71 (-42.1095, 8.9618) -> (-41.402, 11.8065)
  arc A106 (-41.402, 11.8065) -> (-41.3242, 11.5193) centre (-41.1644, 11.7168) ccw
  arc A107 (-41.324, 6.1638) -> (-41.4383, 6.4117) centre (-41.5757, 6.1981) ccw
  arc A108 (-41.6431, 4.9079) -> (-41.4668, 5.1162) centre (-41.7184, 5.1505) ccw
  line L72 (-41.4383, 6.4117) -> (-42.3274, 6.9838)
  line L73 (-42.6529, 4.5945) -> (-41.6431, 4.9079)
  line L74 (-41.4668, 5.1162) -> (-41.324, 6.1638)
  arc A109 (-42.6529, 4.5945) -> (-42.8316, 4.3565) centre (-42.5776, 4.3519) ccw
  line L75 (-42.8316, 4.3565) -> (-42.4358, 7.261)
  arc A110 (-42.4358, 7.261) -> (-42.3274, 6.9838) centre (-42.1899, 7.1974) ccw
  arc A111 (-41.7482, 1.6598) -> (-41.8886, 1.8939) centre (-42.0021, 1.6667) ccw
  arc A112 (-41.9297, 0.3767) -> (-41.7768, 0.6028) centre (-42.0307, 0.6097) ccw
  line L76 (-41.8886, 1.8939) -> (-42.8343, 2.3665)
  line L77 (-42.8996, -0.044) -> (-41.9297, 0.3767)
  line L78 (-41.7768, 0.6028) -> (-41.7482, 1.6598)
  arc A113 (-42.8996, -0.044) -> (-43.0515, -0.3) centre (-42.7985, -0.277) ccw
  line L79 (-43.0515, -0.3) -> (-42.9721, 2.6303)
  arc A114 (-42.9721, 2.6303) -> (-42.8343, 2.3665) centre (-42.7208, 2.5937) ccw
  arc A115 (-41.6829, -2.8637) -> (-41.8478, -2.6462) centre (-41.9361, -2.8843) ccw
  arc A116 (-41.7246, -4.1589) -> (-41.5971, -3.9176) centre (-41.8503, -3.9382) ccw
  line L80 (-41.8478, -2.6462) -> (-42.8391, -2.2786)
  line L81 (-42.6434, -4.682) -> (-41.7246, -4.1589)
  line L82 (-41.5971, -3.9176) -> (-41.6829, -2.8637)
  arc A117 (-42.6434, -4.682) -> (-42.7667, -4.9529) centre (-42.5177, -4.9028) ccw
  line L83 (-42.7667, -4.9529) -> (-43.0046, -2.0312)
  arc A118 (-43.0046, -2.0312) -> (-42.8391, -2.2786) centre (-42.7508, -2.0404) ccw
  arc A119 (-41.129, -7.3536) -> (-41.3164, -7.1552) centre (-41.3784, -7.4015) ccw
  arc A120 (-41.0304, -8.6458) -> (-40.9297, -8.392) centre (-41.1792, -8.4399) ccw
  line L84 (-41.3164, -7.1552) -> (-42.3416, -6.897)
  line L85 (-41.8872, -9.2651) -> (-41.0304, -8.6458)
  line L86 (-40.9297, -8.392) -> (-41.129, -7.3536)
  arc A121 (-41.8872, -9.2651) -> (-41.9805, -9.5478) centre (-41.7384, -9.471) ccw
  line L87 (-41.9805, -9.5478) -> (-42.5329, -6.6689)
  arc A122 (-42.5329, -6.6689) -> (-42.3416, -6.897) centre (-42.2796, -6.6506) ccw
  arc A123 (-40.0928, -11.7574) -> (-40.3006, -11.5803) centre (-40.3356, -11.8319) ccw
  arc A124 (-39.8551, -13.0312) -> (-39.7824, -12.7681) centre (-40.0253, -12.8427) ccw
  line L88 (-40.3006, -11.5803) -> (-41.3477, -11.4345)
  line L89 (-40.6399, -13.7396) -> (-39.8551, -13.0312)
  line L90 (-39.7824, -12.7681) -> (-40.0928, -11.7574)
  arc A125 (-40.6399, -13.7396) -> (-40.7021, -14.0307) centre (-40.4697, -13.9282) ccw
  line L91 (-40.7021, -14.0307) -> (-41.5625, -11.2285)
  arc A126 (-41.5625, -11.2285) -> (-41.3477, -11.4345) centre (-41.3127, -11.1829) ccw
  arc A127 (-38.5866, -16.0232) -> (-38.8123, -15.8697) centre (-38.8199, -16.1236) ccw
  arc A128 (-38.2125, -17.2639) -> (-38.1688, -16.9945) centre (-38.4021, -17.0949) ccw
  line L92 (-38.8123, -15.8697) -> (-39.869, -15.8379)
  line L93 (-38.9162, -18.053) -> (-38.2125, -17.2639)
  line L94 (-38.1688, -16.9945) -> (-38.5866, -16.0232)
  arc A129 (-38.9162, -18.053) -> (-38.9465, -18.3491) centre (-38.7266, -18.2221) ccw
  line L95 (-38.9465, -18.3491) -> (-40.1049, -15.6563)
  arc A130 (-40.1049, -15.6563) -> (-39.869, -15.8379) centre (-39.8614, -15.584) ccw
  arc A131 (-36.628, -20.1012) -> (-36.8689, -19.973) centre (-36.8491, -20.2262) ccw
  arc A132 (-36.1219, -21.2942) -> (-36.1076, -21.0217) centre (-36.3287, -21.1467) ccw
  line L96 (-36.8689, -19.973) -> (-37.9229, -20.0557)
  line L97 (-36.7362, -22.1548) -> (-36.1219, -21.2942)
  line L98 (-36.1076, -21.0217) -> (-36.628, -20.1012)
  arc A133 (-36.7362, -22.1548) -> (-36.7343, -22.4524) centre (-36.5294, -22.3023) ccw
  line L99 (-36.7343, -22.4524) -> (-38.177, -19.9007)
  arc A134 (-38.177, -19.9007) -> (-37.9229, -20.0557) centre (-37.9428, -19.8024) ccw
  arc A135 (-34.2399, -23.9436) -> (-34.4933, -23.8422) centre (-34.4462, -24.0918) ccw
  arc A136 (-33.6079, -25.0749) -> (-33.6231, -24.8023) centre (-33.8294, -24.9505) ccw
  line L100 (-34.4933, -23.8422) -> (-35.5322, -24.0383)
  line L101 (-34.1255, -25.9968) -> (-33.6079, -25.0749)
  line L102 (-33.6231, -24.8023) -> (-34.2399, -23.9436)
  arc A137 (-34.1255, -25.9968) -> (-34.0915, -26.2925) centre (-33.904, -26.1211) ccw
  line L103 (-34.0915, -26.2925) -> (-35.8016, -23.9117)
  arc A138 (-35.8016, -23.9117) -> (-35.5322, -24.0383) centre (-35.5794, -23.7887) ccw
  arc A139 (-31.4504, -27.5052) -> (-31.7133, -27.4318) centre (-31.6395, -27.6748) ccw
  arc A140 (-30.6998, -28.5615) -> (-30.7444, -28.2922) centre (-30.9334, -28.4619) ccw
  line L104 (-31.7133, -27.4318) -> (-32.725, -27.7391)
  line L105 (-31.1147, -29.534) -> (-30.6998, -28.5615)
  line L106 (-30.7444, -28.2922) -> (-31.4504, -27.5052)
  arc A141 (-31.1147, -29.534) -> (-31.0489, -29.8243) centre (-30.881, -29.6337) ccw
  line L107 (-31.0489, -29.8243) -> (-33.0064, -27.6423)
  arc A142 (-33.0064, -27.6423) -> (-32.725, -27.7391) centre (-32.7988, -27.496) ccw
  arc A143 (-28.2922, -30.7444) -> (-28.5615, -30.6998) centre (-28.4619, -30.9334) ccw
  arc A144 (-27.4318, -31.7133) -> (-27.5052, -31.4504) centre (-27.6748, -31.6395) ccw
  line L108 (-28.5615, -30.6998) -> (-29.534, -31.1147)
  line L109 (-27.7391, -32.725) -> (-27.4318, -31.7133)
  line L110 (-27.5052, -31.4504) -> (-28.2922, -30.7444)
  arc A145 (-27.7391, -32.725) -> (-27.6423, -33.0064) centre (-27.496, -32.7988) ccw
  line L111 (-27.6423, -33.0064) -> (-29.8243, -31.0489)
  arc A146 (-29.8243, -31.0489) -> (-29.534, -31.1147) centre (-29.6337, -30.881) ccw
  arc A147 (-24.8023, -33.6231) -> (-25.0749, -33.6079) centre (-24.9505, -33.8294) ccw
  arc A148 (-23.8422, -34.4933) -> (-23.9436, -34.2399) centre (-24.0918, -34.4462) ccw
  line L112 (-25.0749, -33.6079) -> (-25.9968, -34.1255)
  line L113 (-24.0383, -35.5322) -> (-23.8422, -34.4933)
  line L114 (-23.9436, -34.2399) -> (-24.8023, -33.6231)
  arc A149 (-24.0383, -35.5322) -> (-23.9117, -35.8016) centre (-23.7887, -35.5794) ccw
  line L115 (-23.9117, -35.8016) -> (-26.2925, -34.0915)
  arc A150 (-26.2925, -34.0915) -> (-25.9968, -34.1255) centre (-26.1211, -33.904) ccw
  arc A151 (-21.0217, -36.1076) -> (-21.2942, -36.1219) centre (-21.1467, -36.3287) ccw
  arc A152 (-19.973, -36.8689) -> (-20.1012, -36.628) centre (-20.2262, -36.8491) ccw
  line L116 (-21.2942, -36.1219) -> (-22.1548, -36.7362)
  line L117 (-20.0557, -37.9229) -> (-19.973, -36.8689)
  line L118 (-20.1012, -36.628) -> (-21.0217, -36.1076)
  arc A153 (-20.0557, -37.9229) -> (-19.9007, -38.177) centre (-19.8024, -37.9428) ccw
  line L119 (-19.9007, -38.177) -> (-22.4524, -36.7343)
  arc A154 (-22.4524, -36.7343) -> (-22.1548, -36.7362) centre (-22.3023, -36.5294) ccw
  arc A155 (-16.9945, -38.1688) -> (-17.2639, -38.2125) centre (-17.0949, -38.4021) ccw
  arc A156 (-15.8697, -38.8123) -> (-16.0232, -38.5866) centre (-16.1236, -38.8199) ccw
  line L120 (-17.2639, -38.2125) -> (-18.053, -38.9162)
  line L121 (-15.8379, -39.869) -> (-15.8697, -38.8123)
  line L122 (-16.0232, -38.5866) -> (-16.9945, -38.1688)
  arc A157 (-15.8379, -39.869) -> (-15.6563, -40.1049) centre (-15.584, -39.8614) ccw
  line L123 (-15.6563, -40.1049) -> (-18.3491, -38.9465)
  arc A158 (-18.3491, -38.9465) -> (-18.053, -38.9162) centre (-18.2221, -38.7266) ccw
  arc A159 (-12.7681, -39.7824) -> (-13.0312, -39.8551) centre (-12.8427, -40.0253) ccw
  arc A160 (-11.5803, -40.3006) -> (-11.7574, -40.0928) centre (-11.8319, -40.3356) ccw
  line L124 (-13.0312, -39.8551) -> (-13.7396, -40.6399)
  line L125 (-11.4345, -41.3477) -> (-11.5803, -40.3006)
  line L126 (-11.7574, -40.0928) -> (-12.7681, -39.7824)
  arc A161 (-11.4345, -41.3477) -> (-11.2285, -41.5625) centre (-11.1829, -41.3127) ccw
  line L127 (-11.2285, -41.5625) -> (-14.0307, -40.7021)
  arc A162 (-14.0307, -40.7021) -> (-13.7396, -40.6399) centre (-13.9282, -40.4697) ccw
  arc A163 (-8.392, -40.9297) -> (-8.6458, -41.0304) centre (-8.4399, -41.1792) ccw
  arc A164 (-7.1552, -41.3164) -> (-7.3536, -41.129) centre (-7.4015, -41.3784) ccw
  line L128 (-8.6458, -41.0304) -> (-9.2651, -41.8872)
  line L129 (-6.897, -42.3416) -> (-7.1552, -41.3164)
  line L130 (-7.3536, -41.129) -> (-8.392, -40.9297)
  arc A165 (-6.897, -42.3416) -> (-6.6689, -42.5329) centre (-6.6506, -42.2796) ccw
  line L131 (-6.6689, -42.5329) -> (-9.5478, -41.9805)
  arc A166 (-9.5478, -41.9805) -> (-9.2651, -41.8872) centre (-9.471, -41.7384) ccw
  arc A167 (-3.9176, -41.5971) -> (-4.1589, -41.7246) centre (-3.9382, -41.8503) ccw
  arc A168 (-2.6462, -41.8478) -> (-2.8637, -41.6829) centre (-2.8843, -41.9361) ccw
  line L132 (-4.1589, -41.7246) -> (-4.682, -42.6434)
  line L133 (-2.2786, -42.8391) -> (-2.6462, -41.8478)
  line L134 (-2.8637, -41.6829) -> (-3.9176, -41.5971)
  arc A169 (-2.2786, -42.8391) -> (-2.0312, -43.0046) centre (-2.0404, -42.7508) ccw
  line L135 (-2.0312, -43.0046) -> (-4.9529, -42.7667)
  arc A170 (-4.9529, -42.7667) -> (-4.682, -42.6434) centre (-4.9028, -42.5177) ccw
  arc A171 (0.6028, -41.7768) -> (0.3767, -41.9297) centre (0.6097, -42.0307) ccw
  arc A172 (1.8939, -41.8886) -> (1.6598, -41.7482) centre (1.6667, -42.0021) ccw
  line L136 (0.3767, -41.9297) -> (-0.044, -42.8996)
  line L137 (2.3665, -42.8343) -> (1.8939, -41.8886)
  line L138 (1.6598, -41.7482) -> (0.6028, -41.7768)
  arc A173 (2.3665, -42.8343) -> (2.6303, -42.9721) centre (2.5937, -42.7208) ccw
  line L139 (2.6303, -42.9721) -> (-0.3, -43.0515)
  arc A174 (-0.3, -43.0515) -> (-0.044, -42.8996) centre (-0.277, -42.7985) ccw
  arc A175 (5.1162, -41.4668) -> (4.9079, -41.6431) centre (5.1505, -41.7184) ccw
  arc A176 (6.4117, -41.4383) -> (6.1638, -41.324) centre (6.1981, -41.5757) ccw
  line L140 (4.9079, -41.6431) -> (4.5945, -42.6529)
  line L141 (6.9838, -42.3274) -> (6.4117, -41.4383)
  line L142 (6.1638, -41.324) -> (5.1162, -41.4668)
  arc A177 (6.9838, -42.3274) -> (7.261, -42.4358) centre (7.1974, -42.1899) ccw
  line L143 (7.261, -42.4358) -> (4.3565, -42.8316)
  arc A178 (4.3565, -42.8316) -> (4.5945, -42.6529) centre (4.3519, -42.5776) ccw
  arc A179 (9.5695, -40.6705) -> (9.3815, -40.8684) centre (9.6308, -40.917) ccw
  arc A180 (10.8544, -40.5021) -> (10.5956, -40.4153) centre (10.6569, -40.6618) ccw
  line L144 (9.3815, -40.8684) -> (9.1792, -41.9061)
  line L145 (11.5193, -41.3242) -> (10.8544, -40.5021)
  line L146 (10.5956, -40.4153) -> (9.5695, -40.6705)
  arc A181 (11.5193, -41.3242) -> (11.8065, -41.402) centre (11.7168, -41.1644) ccw
  line L147 (11.8065, -41.402) -> (8.9618, -42.1095)
  arc A182 (8.9618, -42.1095) -> (9.1792, -41.9061) centre (8.9299, -41.8575) ccw
  arc A183 (13.9107, -39.3975) -> (13.7452, -39.6145) centre (13.9983, -39.6359) ccw
  arc A184 (15.1698, -39.0911) -> (14.9032, -39.0328) centre (14.9908, -39.2713) ccw
  line L148 (13.7452, -39.6145) -> (13.6562, -40.668)
  line L149 (15.9197, -39.8365) -> (15.1698, -39.0911)
  line L150 (14.9032, -39.0328) -> (13.9107, -39.3975)
  arc A185 (15.9197, -39.8365) -> (16.2137, -39.8828) centre (16.0987, -39.6563) ccw
  line L151 (16.2137, -39.8828) -> (13.4621, -40.8937)
  arc A186 (13.4621, -40.8937) -> (13.6562, -40.668) centre (13.4031, -40.6466) ccw
  arc A187 (18.0888, -37.6625) -> (17.9477, -37.8962) centre (18.2016, -37.8901) ccw
  arc A188 (19.3074, -37.2218) -> (19.036, -37.1927) centre (19.1489, -37.4203) ccw
  line L152 (17.9477, -37.8962) -> (17.9731, -38.9531)
  line L153 (20.1334, -37.8817) -> (19.3074, -37.2218)
  line L154 (19.036, -37.1927) -> (18.0888, -37.6625)
  arc A189 (20.1334, -37.8817) -> (20.4307, -37.896) centre (20.292, -37.6833) ccw
  line L155 (20.4307, -37.896) -> (17.8046, -39.1985)
  arc A190 (17.8046, -39.1985) -> (17.9731, -38.9531) centre (17.7192, -38.9592) ccw
  arc A191 (22.0548, -35.486) -> (21.9398, -35.7335) centre (22.1916, -35.7) ccw
  arc A192 (23.2186, -34.9161) -> (22.9457, -34.9165) centre (23.0825, -35.1305) ccw
  line L156 (21.9398, -35.7335) -> (22.0794, -36.7815)
  line L157 (24.1111, -35.4828) -> (23.2186, -34.9161)
  line L158 (22.9457, -34.9165) -> (22.0548, -35.486)
  arc A193 (24.1111, -35.4828) -> (24.4082, -35.4649) centre (24.2473, -35.2684) ccw
  line L159 (24.4082, -35.4649) -> (21.9383, -37.0437)
  arc A194 (21.9383, -37.0437) -> (22.0794, -36.7815) centre (21.8276, -36.8151) ccw
  arc A195 (25.7622, -32.8934) -> (25.6746, -33.152) centre (25.9213, -33.0914) ccw
  arc A196 (26.8576, -32.2011) -> (26.5863, -32.231) centre (26.7454, -32.429) ccw
  line L160 (25.6746, -33.152) -> (25.9267, -34.1787)
  line L161 (27.8062, -32.668) -> (26.8576, -32.2011)
  line L162 (26.5863, -32.231) -> (25.7622, -32.8934)
  arc A197 (27.8062, -32.668) -> (28.0996, -32.618) centre (27.9183, -32.4401) ccw
  line L163 (28.0996, -32.618) -> (25.8149, -34.4545)
  arc A198 (25.8149, -34.4545) -> (25.9267, -34.1787) centre (25.68, -34.2393) ccw
  arc A199 (29.1676, -29.9152) -> (29.1085, -30.1817) centre (29.3472, -30.0948) ccw
  arc A200 (30.1817, -29.1085) -> (29.9152, -29.1676) centre (30.0948, -29.3472) ccw
  line L164 (29.1085, -30.1817) -> (29.4701, -31.1752)
  line L165 (31.1752, -29.4701) -> (30.1817, -29.1085)
  line L166 (29.9152, -29.1676) -> (29.1676, -29.9152)
  arc A201 (31.1752, -29.4701) -> (31.4615, -29.3887) centre (31.2621, -29.2314) ccw
  line L167 (31.4615, -29.3887) -> (29.3887, -31.4615)
  arc A202 (29.3887, -31.4615) -> (29.4701, -31.1752) centre (29.2314, -31.2621) ccw
  arc A203 (32.231, -26.5863) -> (32.2011, -26.8576) centre (32.429, -26.7454) ccw
  arc A204 (33.152, -25.6746) -> (32.8934, -25.7622) centre (33.0914, -25.9213) ccw
  line L168 (32.2011, -26.8576) -> (32.668, -27.8062)
  line L169 (34.1787, -25.9267) -> (33.152, -25.6746)
  line L170 (32.8934, -25.7622) -> (32.231, -26.5863)
  arc A205 (34.1787, -25.9267) -> (34.4545, -25.8149) centre (34.2393, -25.68) ccw
  line L171 (34.4545, -25.8149) -> (32.618, -28.0996)
  arc A206 (32.618, -28.0996) -> (32.668, -27.8062) centre (32.4401, -27.9183) ccw
  arc A207 (34.9165, -22.9457) -> (34.9161, -23.2186) centre (35.1305, -23.0825) ccw
  arc A208 (35.7335, -21.9398) -> (35.486, -22.0548) centre (35.7, -22.1916) ccw
  line L172 (34.9161, -23.2186) -> (35.4828, -24.1111)
  line L173 (36.7815, -22.0794) -> (35.7335, -21.9398)
  line L174 (35.486, -22.0548) -> (34.9165, -22.9457)
  arc A209 (36.7815, -22.0794) -> (37.0437, -21.9383) centre (36.8151, -21.8276) ccw
  line L175 (37.0437, -21.9383) -> (35.4649, -24.4082)
  arc A210 (35.4649, -24.4082) -> (35.4828, -24.1111) centre (35.2684, -24.2473) ccw
  arc A211 (37.1927, -19.036) -> (37.2218, -19.3074) centre (37.4203, -19.1489) ccw
  arc A212 (37.8962, -17.9477) -> (37.6625, -18.0888) centre (37.8901, -18.2016) ccw
  line L176 (37.2218, -19.3074) -> (37.8817, -20.1334)
  line L177 (38.9531, -17.9731) -> (37.8962, -17.9477)
  line L178 (37.6625, -18.0888) -> (37.1927, -19.036)
  arc A213 (38.9531, -17.9731) -> (39.1985, -17.8046) centre (38.9592, -17.7192) ccw
  line L179 (39.1985, -17.8046) -> (37.896, -20.4307)
  arc A214 (37.896, -20.4307) -> (37.8817, -20.1334) centre (37.6833, -20.292) ccw
  arc A215 (39.0328, -14.9032) -> (39.0911, -15.1698) centre (39.2713, -14.9908) ccw
  arc A216 (39.6145, -13.7452) -> (39.3975, -13.9107) centre (39.6359, -13.9983) ccw
  line L180 (39.0911, -15.1698) -> (39.8365, -15.9197)
  line L181 (40.668, -13.6562) -> (39.6145, -13.7452)
  line L182 (39.3975, -13.9107) -> (39.0328, -14.9032)
  arc A217 (40.668, -13.6562) -> (40.8937, -13.4621) centre (40.6466, -13.4031) ccw
  line L183 (40.8937, -13.4621) -> (39.8828, -16.2137)
  arc A218 (39.8828, -16.2137) -> (39.8365, -15.9197) centre (39.6563, -16.0987) ccw
  arc A219 (40.4153, -10.5956) -> (40.5021, -10.8544) centre (40.6618, -10.6569) ccw
  arc A220 (40.8684, -9.3815) -> (40.6705, -9.5695) centre (40.917, -9.6308) ccw
  line L184 (40.5021, -10.8544) -> (41.3242, -11.5193)
  line L185 (41.9061, -9.1792) -> (40.8684, -9.3815)
  line L186 (40.6705, -9.5695) -> (40.4153, -10.5956)
  arc A221 (41.9061, -9.1792) -> (42.1095, -8.9618) centre (41.8575, -8.9299) ccw
  line L187 (42.1095, -8.9618) -> (41.402, -11.8065)
  arc A222 (41.402, -11.8065) -> (41.3242, -11.5193) centre (41.1644, -11.7168) ccw
  arc A223 (41.324, -6.1638) -> (41.4383, -6.4117) centre (41.5757, -6.1981) ccw
  arc A224 (41.6431, -4.9079) -> (41.4668, -5.1162) centre (41.7184, -5.1505) ccw
  line L188 (41.4383, -6.4117) -> (42.3274, -6.9838)
  line L189 (42.6529, -4.5945) -> (41.6431, -4.9079)
  line L190 (41.4668, -5.1162) -> (41.324, -6.1638)
  arc A225 (42.6529, -4.5945) -> (42.8316, -4.3565) centre (42.5776, -4.3519) ccw
  line L191 (42.8316, -4.3565) -> (42.4358, -7.261)
  arc A226 (42.4358, -7.261) -> (42.3274, -6.9838) centre (42.1899, -7.1974) ccw
  arc A227 (41.7482, -1.6598) -> (41.8886, -1.8939) centre (42.0021, -1.6667) ccw
  arc A228 (41.9297, -0.3767) -> (41.7768, -0.6028) centre (42.0307, -0.6097) ccw
  line L192 (41.8886, -1.8939) -> (42.8343, -2.3665)
  line L193 (42.8996, 0.044) -> (41.9297, -0.3767)
  line L194 (41.7768, -0.6028) -> (41.7482, -1.6598)
  arc A229 (42.8996, 0.044) -> (43.0515, 0.3) centre (42.7985, 0.277) ccw
  line L195 (43.0515, 0.3) -> (42.9721, -2.6303)
  arc A230 (42.9721, -2.6303) -> (42.8343, -2.3665) centre (42.7208, -2.5937) ccw
  arc A231 (41.6829, 2.8637) -> (41.8478, 2.6462) centre (41.9361, 2.8843) ccw
  arc A232 (41.7246, 4.1589) -> (41.5971, 3.9176) centre (41.8503, 3.9382) ccw
  line L196 (41.8478, 2.6462) -> (42.8391, 2.2786)
  line L197 (42.6434, 4.682) -> (41.7246, 4.1589)
  line L198 (41.5971, 3.9176) -> (41.6829, 2.8637)
  arc A233 (42.6434, 4.682) -> (42.7667, 4.9529) centre (42.5177, 4.9028) ccw
  line L199 (42.7667, 4.9529) -> (43.0046, 2.0312)
  arc A234 (43.0046, 2.0312) -> (42.8391, 2.2786) centre (42.7508, 2.0404) ccw
  arc A235 (41.129, 7.3536) -> (41.3164, 7.1552) centre (41.3784, 7.4015) ccw
  arc A236 (41.0304, 8.6458) -> (40.9297, 8.392) centre (41.1792, 8.4399) ccw
  line L200 (41.3164, 7.1552) -> (42.3416, 6.897)
  line L201 (41.8872, 9.2651) -> (41.0304, 8.6458)
  line L202 (40.9297, 8.392) -> (41.129, 7.3536)
  arc A237 (41.8872, 9.2651) -> (41.9805, 9.5478) centre (41.7384, 9.471) ccw
  line L203 (41.9805, 9.5478) -> (42.5329, 6.6689)
  arc A238 (42.5329, 6.6689) -> (42.3416, 6.897) centre (42.2796, 6.6506) ccw
  arc A239 (40.0928, 11.7574) -> (40.3006, 11.5803) centre (40.3356, 11.8319) ccw
  arc A240 (39.8551, 13.0312) -> (39.7824, 12.7681) centre (40.0253, 12.8427) ccw
  line L204 (40.3006, 11.5803) -> (41.3477, 11.4345)
  line L205 (40.6399, 13.7396) -> (39.8551, 13.0312)
  line L206 (39.7824, 12.7681) -> (40.0928, 11.7574)
  arc A241 (40.6399, 13.7396) -> (40.7021, 14.0307) centre (40.4697, 13.9282) ccw
  line L207 (40.7021, 14.0307) -> (41.5625, 11.2285)
  arc A242 (41.5625, 11.2285) -> (41.3477, 11.4345) centre (41.3127, 11.1829) ccw
  arc A243 (38.5866, 16.0232) -> (38.8123, 15.8697) centre (38.8199, 16.1236) ccw
  arc A244 (38.2125, 17.2639) -> (38.1688, 16.9945) centre (38.4021, 17.0949) ccw
  line L208 (38.8123, 15.8697) -> (39.869, 15.8379)
  line L209 (38.9162, 18.053) -> (38.2125, 17.2639)
  line L210 (38.1688, 16.9945) -> (38.5866, 16.0232)
  arc A245 (38.9162, 18.053) -> (38.9465, 18.3491) centre (38.7266, 18.2221) ccw
  line L211 (38.9465, 18.3491) -> (40.1049, 15.6563)
  arc A246 (40.1049, 15.6563) -> (39.869, 15.8379) centre (39.8614, 15.584) ccw
  arc A247 (36.628, 20.1012) -> (36.8689, 19.973) centre (36.8491, 20.2262) ccw
  arc A248 (36.1219, 21.2942) -> (36.1076, 21.0217) centre (36.3287, 21.1467) ccw
  line L212 (36.8689, 19.973) -> (37.9229, 20.0557)
  line L213 (36.7362, 22.1548) -> (36.1219, 21.2942)
  line L214 (36.1076, 21.0217) -> (36.628, 20.1012)
  arc A249 (36.7362, 22.1548) -> (36.7343, 22.4524) centre (36.5294, 22.3023) ccw
  line L215 (36.7343, 22.4524) -> (38.177, 19.9007)
  arc A250 (38.177, 19.9007) -> (37.9229, 20.0557) centre (37.9428, 19.8024) ccw
  arc A251 (34.2399, 23.9436) -> (34.4933, 23.8422) centre (34.4462, 24.0918) ccw
  arc A252 (33.6079, 25.0749) -> (33.6231, 24.8023) centre (33.8294, 24.9505) ccw
  line L216 (34.4933, 23.8422) -> (35.5322, 24.0383)
  line L217 (34.1255, 25.9968) -> (33.6079, 25.0749)
  line L218 (33.6231, 24.8023) -> (34.2399, 23.9436)
  arc A253 (34.1255, 25.9968) -> (34.0915, 26.2925) centre (33.904, 26.1211) ccw
  line L219 (34.0915, 26.2925) -> (35.8016, 23.9117)
  arc A254 (35.8016, 23.9117) -> (35.5322, 24.0383) centre (35.5794, 23.7887) ccw
  arc A255 (31.4504, 27.5052) -> (31.7133, 27.4318) centre (31.6395, 27.6748) ccw
  arc A256 (30.6998, 28.5615) -> (30.7444, 28.2922) centre (30.9334, 28.4619) ccw
  line L220 (31.7133, 27.4318) -> (32.725, 27.7391)
  line L221 (31.1147, 29.534) -> (30.6998, 28.5615)
  line L222 (30.7444, 28.2922) -> (31.4504, 27.5052)
  arc A257 (31.1147, 29.534) -> (31.0489, 29.8243) centre (30.881, 29.6337) ccw
  line L223 (31.0489, 29.8243) -> (33.0064, 27.6423)
  arc A258 (33.0064, 27.6423) -> (32.725, 27.7391) centre (32.7988, 27.496) ccw
  arc A259 (28.2922, 30.7444) -> (28.5615, 30.6998) centre (28.4619, 30.9334) ccw
  arc A260 (27.4318, 31.7133) -> (27.5052, 31.4504) centre (27.6748, 31.6395) ccw
  line L224 (28.5615, 30.6998) -> (29.534, 31.1147)
  line L225 (27.7391, 32.725) -> (27.4318, 31.7133)
  line L226 (27.5052, 31.4504) -> (28.2922, 30.7444)
  arc A261 (27.7391, 32.725) -> (27.6423, 33.0064) centre (27.496, 32.7988) ccw
  line L227 (27.6423, 33.0064) -> (29.8243, 31.0489)
  arc A262 (29.8243, 31.0489) -> (29.534, 31.1147) centre (29.6337, 30.881) ccw
  arc A263 (24.8023, 33.6231) -> (25.0749, 33.6079) centre (24.9505, 33.8294) ccw
  arc A264 (23.8422, 34.4933) -> (23.9436, 34.2399) centre (24.0918, 34.4462) ccw
  line L228 (25.0749, 33.6079) -> (25.9968, 34.1255)
  line L229 (24.0383, 35.5322) -> (23.8422, 34.4933)
  line L230 (23.9436, 34.2399) -> (24.8023, 33.6231)
  arc A265 (24.0383, 35.5322) -> (23.9117, 35.8016) centre (23.7887, 35.5794) ccw
  line L231 (23.9117, 35.8016) -> (26.2925, 34.0915)
  arc A266 (26.2925, 34.0915) -> (25.9968, 34.1255) centre (26.1211, 33.904) ccw
  arc A267 (21.0217, 36.1076) -> (21.2942, 36.1219) centre (21.1467, 36.3287) ccw
  arc A268 (19.973, 36.8689) -> (20.1012, 36.628) centre (20.2262, 36.8491) ccw
  line L232 (21.2942, 36.1219) -> (22.1548, 36.7362)
  line L233 (20.0557, 37.9229) -> (19.973, 36.8689)
  line L234 (20.1012, 36.628) -> (21.0217, 36.1076)
  arc A269 (20.0557, 37.9229) -> (19.9007, 38.177) centre (19.8024, 37.9428) ccw
  line L235 (19.9007, 38.177) -> (22.4524, 36.7343)
  arc A270 (22.4524, 36.7343) -> (22.1548, 36.7362) centre (22.3023, 36.5294) ccw
  arc A271 (16.9945, 38.1688) -> (17.2639, 38.2125) centre (17.0949, 38.4021) ccw
  arc A272 (15.8697, 38.8123) -> (16.0232, 38.5866) centre (16.1236, 38.8199) ccw
  line L236 (17.2639, 38.2125) -> (18.053, 38.9162)
  line L237 (15.8379, 39.869) -> (15.8697, 38.8123)
  line L238 (16.0232, 38.5866) -> (16.9945, 38.1688)
  arc A273 (15.8379, 39.869) -> (15.6563, 40.1049) centre (15.584, 39.8614) ccw
  line L239 (15.6563, 40.1049) -> (18.3491, 38.9465)
  arc A274 (18.3491, 38.9465) -> (18.053, 38.9162) centre (18.2221, 38.7266) ccw
  arc A275 (12.7681, 39.7824) -> (13.0312, 39.8551) centre (12.8427, 40.0253) ccw
  arc A276 (11.5803, 40.3006) -> (11.7574, 40.0928) centre (11.8319, 40.3356) ccw
  line L240 (13.0312, 39.8551) -> (13.7396, 40.6399)
  line L241 (11.4345, 41.3477) -> (11.5803, 40.3006)
  line L242 (11.7574, 40.0928) -> (12.7681, 39.7824)
  arc A277 (11.4345, 41.3477) -> (11.2285, 41.5625) centre (11.1829, 41.3127) ccw
  line L243 (11.2285, 41.5625) -> (14.0307, 40.7021)
  arc A278 (14.0307, 40.7021) -> (13.7396, 40.6399) centre (13.9282, 40.4697) ccw
  arc A279 (8.392, 40.9297) -> (8.6458, 41.0304) centre (8.4399, 41.1792) ccw
  arc A280 (7.1552, 41.3164) -> (7.3536, 41.129) centre (7.4015, 41.3784) ccw
  line L244 (8.6458, 41.0304) -> (9.2651, 41.8872)
  line L245 (6.897, 42.3416) -> (7.1552, 41.3164)
  line L246 (7.3536, 41.129) -> (8.392, 40.9297)
  arc A281 (6.897, 42.3416) -> (6.6689, 42.5329) centre (6.6506, 42.2796) ccw
  line L247 (6.6689, 42.5329) -> (9.5478, 41.9805)
  arc A282 (9.5478, 41.9805) -> (9.2651, 41.8872) centre (9.471, 41.7384) ccw
  arc A283 (3.9176, 41.5971) -> (4.1589, 41.7246) centre (3.9382, 41.8503) ccw
  arc A284 (2.6462, 41.8478) -> (2.8637, 41.6829) centre (2.8843, 41.9361) ccw
  line L248 (4.1589, 41.7246) -> (4.682, 42.6434)
  line L249 (2.2786, 42.8391) -> (2.6462, 41.8478)